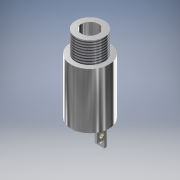
# Autodesk Inventor part: MJ-074N
Saved by Autodesk Inventor 2016 (Build 200138000, 138)
## iProperties
Created: 2016-06-17
Part Number: MJ-074N
Material: Nickel-Copper Alloy 400
Document SubType Name: Modeling
Designer: Tyler
Density: 8.83 g/cm^3
Appearance: Chrome - Polished
Stock Number: AV15152
Author: Tyler
Autodesk Inventor part; units mm, degrees
ref_plane "YZ Plane" through (0, 0, 0) normal (1, 0, 0) x (0, 1, 0)
ref_plane "XZ Plane" through (0, 0, 0) normal (0, 1, 0) x (-1, 0, 0)
ref_plane "XY Plane" through (0, 0, 0) normal (0, 0, 1) x (1, 0, 0)
sketch "Sketch1" plane through (0, 0, 0) normal (0, 0, 1) x (1, 0, 0)
  circle A0 centre (0, 0) radius 4
  dimension "d0" = 8
  constraints: 1 centre point, 1 coincident
  measures "d0" diameter of A0
extrude "Extrusion1" add sketch "Sketch1" against normal blind 11.7
sketch "Sketch2" plane through (0, 0, 0) normal (0, 0, 1) x (1, 0, 0)
  circle A0 centre (0, 0) radius 4 projected
  circle A1 centre (0, 0) radius 3
  dimension "d3" = 6
  constraints: 1 centre point, 1 coincident
  measures "d3" diameter of A1
extrude "Extrusion2" add sketch "Sketch2" along normal blind 4.5 contours A1
thread "Thread1" size "M6x0.5" class "6g" standard "ANSI Metric M Profile" full length
sketch "Sketch3" plane through (0, 0, 4.5) normal (0, 0, 1) x (1, 0, 0)
  circle A0 centre (0, 0) radius 3 projected
  circle A1 centre (0, 0) radius 1.8
  dimension "d8" = 3.6
  constraints: 1 centre point, 1 coincident
  measures "d8" diameter of A1
extrude "Extrusion3" cut sketch "Sketch3" against normal blind 15 contours A1
sketch "Sketch4" plane through (0, 0, -11.7) normal (0, 0, -1) x (-1, 0, 0)
  circle A0 centre (0, 0) radius 4 construction
  line L0 (0, 0) -> (0, 2.7273) construction
  line L1 (-2.5, 1) -> (-2, 1)
  line L2 (-2, 1) -> (-2, -1)
  line L3 (-2, -1) -> (-2.5, -1)
  line L4 (-2.5, -1) -> (-2.5, 1)
  line L5 (2.5, 1) -> (2, 1)
  line L6 (2, 1) -> (2, -1)
  line L7 (2, -1) -> (2.5, -1)
  line L8 (2.5, -1) -> (2.5, 1)
  dimension "d11" = 2
  dimension "d12" = 0.5
  dimension "d13" = 2
  dimension "d14" = 1
  constraints: 18 end point, 4 symmetric about line, 2 parallel, 1 horizontal, 1 perpendicular, 1 vertical
  measures "d11" distance of L3.end L1.start
  measures "d12" distance of L1.start L1.end
  measures "d13" distance between parallel lines of L2 L0
  measures "d14" distance from line of L0.start L1
extrude "Extrusion4" add sketch "Sketch4" along normal blind 3
sketch "Sketch5" plane through (0, 0, -11.7) normal (0, 0, -1) x (-1, 0, 0)
  circle A0 centre (0, 0) radius 4 projected
  line L0 (-1, 2) -> (1, 2)
  line L1 (1, 2) -> (1, 2.5)
  line L2 (1, 2.5) -> (-1, 2.5)
  line L3 (-1, 2.5) -> (-1, 2)
  line L4 (-1, 2) -> (1, 2.5) construction
  line L5 (1, 2) -> (-1, 2.5) construction
  point P0 (0, 2.25)
  dimension "d17" = 2
  dimension "d18" = 0.5
  dimension "d19" = 2
  dimension "d20" = 1
  constraints: 12 end point, 2 midpoint, 2 parallel, 1 horizontal, 1 perpendicular
  measures "d17" distance of L2.end L1.end
  measures "d18" distance of L1.end L0.end
  measures "d19" distance from line of A0.centre L0
  measures "d20" distance from line of A0.centre L1
extrude "Extrusion5" add sketch "Sketch5" along normal blind 6.1 contours L3 L2 L1 L0
sketch "Sketch6" plane through (2.5, -1, -11.7) normal (1, 0, 0) x (0, 0, -1)
  line L0 (3, 2) -> (3, 0) projected
  circle A0 centre (2, 1) radius 0.5
  point P0 (-11.7, 1)
  dimension "d23" = 1
  dimension "d24" = 1
  constraints: 1 centre point
  measures "d23" diameter of A0
  measures "d24" distance from line of L0 A0.centre
extrude "Extrusion6" cut sketch "Sketch6" against normal through all
sketch "Sketch7" plane through (-1, 2.5, -11.7) normal (0, 1, 0) x (1, 0, 0)
  line L0 (0, 6.1) -> (2, 6.1) projected
  circle A0 centre (1, 5.1) radius 0.5
  point P0 (1, -11.7)
  dimension "d27" = 1
  dimension "d28" = 1
  constraints: 1 centre point
  measures "d27" diameter of A0
  measures "d28" distance from line of A0.centre L0
extrude "Extrusion7" cut sketch "Sketch7" against normal blind 6.1
sketch "Sketch8" plane through (2.5, -1, -11.7) normal (1, 0, 0) x (0, 0, -1)
  circle A0 centre (2, 1) radius 0.5 projected
sketch "Sketch9" plane through (-1, 2, -11.7) normal (0, -1, 0) x (1, 0, 0)
  circle A0 centre (1, -5.1) radius 0.5 projected
sketch "Sketch10" plane through (-2.5, -1, -11.7) normal (-1, 0, 0) x (0, 0, 1)
  circle A0 centre (-2, 1) radius 0.5 projected
equation "\"d14\" = 0.5 * d11"
equation "\"d20\" = 0.5 * d17"
body "Solid1"
